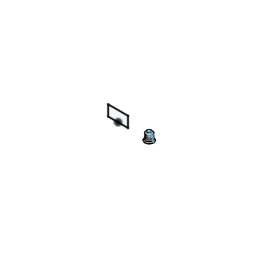
Pin (Autodesk Fusion 360 design; units mm, degrees)
Autodesk Fusion 360 part; units mm, degrees
sketch "Sketch2" plane through (23.0385, 0, 0) normal (1, 0, 0) x (0, 1, 0)
  line L0 (2.9089, 2.85) -> (7.0911, 2.85)
  spline S0 degree 2 poles (6.9365, 3) (7.011, 2.9279) (7.0911, 2.85) knots 0 0 0 0.0233 0.0233 0.0233 weights 1 1.002134 1.00288
  line L1 (6.9365, 3) -> (6.9365, 4)
  spline S1 degree 2 poles (7.4495, 4.5) (7.1645, 4.2208) (6.9365, 4) knots 0 0 0 0.071636 0.071636 0.071636 weights 1 1.006562 1
  line L2 (7.4495, 4.5) -> (7.4495, 4.8082)
  spline S2 degree 2 poles (6.4142, 6) (6.8024, 5.5638) (7.4495, 4.8082) knots 0 0 0 0.157865 0.157865 0.157865 weights 1 1.035276 1
  line L3 (6.4142, 6) -> (3.5858, 6)
  spline S3 degree 2 poles (2.5505, 4.8082) (3.1976, 5.5638) (3.5858, 6) knots 0 0 0 0.157865 0.157865 0.157865 weights 1 1.035276 1
  line L4 (2.5505, 4.8082) -> (2.5505, 4.5)
  spline S4 degree 2 poles (3.0635, 4) (2.8355, 4.2208) (2.5505, 4.5) knots 0 0 0 0.071636 0.071636 0.071636 weights 1 1.006562 1
  line L5 (3.0635, 4) -> (3.0635, 3)
  line L6 (3.0635, 4) -> (3.0635, 5.4041)
  line L7 (6.9365, 4) -> (6.9365, 5.4041)
  line L8 (8.0014, 5.4041) -> (8.0014, 4)
  line L9 (8.0014, 4) -> (6.9365, 4)
  line L10 (3.0635, 4) -> (2.4094, 4)
  line L11 (2.4094, 4) -> (2.4094, 5.4078)
  line L12 (2.4094, 5.4078) -> (3.0635, 5.4041)
  line L13 (6.9365, 5.4041) -> (8.0014, 5.4041)
  spline S5 degree 2 poles (2.9089, 2.85) (2.989, 2.9279) (3.0635, 3) knots 0.048335 0.048335 0.048335 0.071636 0.071636 0.071636 weights 1.00288 1.002134 1
  constraint coincident S4.start L5.start
  constraint coincident S3 L6.end
  constraint parallel L5 L6
  constraint coincident L1.end S1.end
  constraint coincident S2 L7.end
  constraint parallel L1 L7
  constraint parallel L7 L8
  constraint perpendicular L7 L9
  constraint perpendicular L6 L10
  constraint perpendicular L10 L11
  constraint perpendicular L8 L13
sketch "Sketch1" plane through (0, 5, 0) normal (0, 1, 0) x (-1, 0, 0)
  line L0 (-7.5, 0) -> (7.5, 0)
  line L1 (7.5, 0) -> (7.5, 8)
  line L2 (7.5, 8) -> (-7.5, 8)
  line L3 (-7.5, 8) -> (-7.5, 0)
  line L4 (-23.5385, 0) -> (-23.5385, 6)
  line L5 (-23.5385, 6) -> (-25.0385, 6)
  line L6 (-25.0385, 6) -> (-26.0385, 4.8082)
  line L7 (-26.0385, 4.8082) -> (-26.0385, 0.8)
  line L8 (-26.0385, 0.8) -> (-26.8385, 0)
  line L9 (-26.8385, 0) -> (-23.5385, 0)
  line L10 (-26.0385, 4.5) -> (-25.5385, 4)
  line L11 (-25.5385, 4) -> (-25.5385, 3)
  line L12 (-25.5385, 3) -> (-26.0385, 2.5)
  line L13 (-24.0385, 6) -> (-24.0385, 2.4)
  line L14 (-24.0385, 2.4) -> (-23.5385, 2.4)
  line L15 (-23.0385, 6) -> (-23.0385, 2.4)
  line L16 (-23.0385, 2.4) -> (-23.5385, 2.4)
  line L17 (-23.0385, 6) -> (-23.5385, 6)
  dimension "d5" = 6
  dimension "d6" = 5
  dimension "d7" = 3
  dimension "d8" = 6.6
  dimension "d9" = 135
  dimension "d11" = 1
  dimension "d12" = 3
  dimension "d13" = 4
  dimension "d14" = 90
  dimension "d24" = 1
  dimension "d25" = 3.6
  dimension "d31" = 130
  constraint vertical L4
  constraint horizontal L4.start origin
  constraint coincident L4 L5.start
  constraint perpendicular L4 L5
  constraint perpendicular L5 L7
  constraint perpendicular L7 L9
  constraint coincident L4.start L9.end
  constraint coincident L4.end L5.start
  constraint coincident L7 L10.start
  constraint parallel L7 L11
  constraint coincident L7 L12.end
  constraint equal L10 L12
  constraint coincident L5 L13.start
  constraint perpendicular L5 L13
  constraint coincident L4 L14.end
  constraint perpendicular L4 L14
  constraint symmetric L4 L13.start L15.start
  constraint symmetric L4 L13.end L15.end
  constraint symmetric L4 L14.end L16.end
  measures "d5" distance of L4.start L4.end
  measures "d9" angle of L7 L8
  measures "d11" distance of L10.end L11.end
  measures "d12" distance of L9 L11.end
  measures "d14" angle of L10 L12
  measures "d25" distance of L5 L14
  measures "d31" angle of L5 L6
revolve "Revolve1" add sketch "Sketch1" angle 360 about axis through (23.5385, 5, 0) along (0, 0, 1) contours L4 L5 L6 L7 L8 L9 L10 L11 L12 L13 L14 | L4 L5 L13 L14
extrude "Extrude1" [suppressed]
fillet "Fillet1" [suppressed]
extrude "Extrude2" [suppressed]
equation "d8 = 5 mm + ( 2 * 0.8 ) * 1 mm"
named bodies: "pin"
